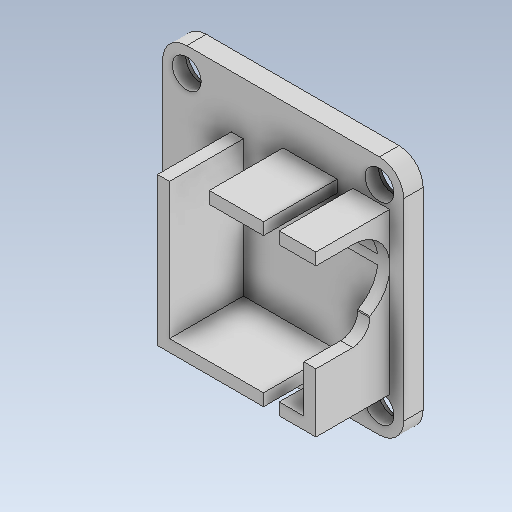
# Autodesk Inventor part: apoio servo
Saved by Autodesk Inventor 2020 (Build 240168000, 168)
## iProperties
Created: 2020-04-22
Part Number: apoio servo
Material: Genérico
Document SubType Name: Modeling
Designer: gi-se
Density: 1 g/cm^3
Appearance: Padrão
Author: gi-se
Autodesk Inventor part; units mm, degrees
ref_plane "YZ Plane" through (0, 0, 0) normal (1, 0, 0) x (0, 1, 0)
ref_plane "XZ Plane" through (0, 0, 0) normal (0, 1, 0) x (-1, 0, 0)
ref_plane "XY Plane" through (0, 0, 0) normal (0, 0, 1) x (1, 0, 0)
sketch "Esboço1" plane through (0, 0, 0) normal (0, 0, 1) x (1, 0, 0)
  circle A0 centre (0, 51.901) radius 2.4 projected
  circle A1 centre (0, 19.901) radius 2.4 projected
  circle A2 centre (-32, 19.901) radius 2.4 projected
  line L0 (-36, 3.901) -> (-36, 51.901) projected
  circle A3 centre (0, 19.901) radius 4
  circle A4 centre (0, 51.901) radius 4
  circle A5 centre (-32, 19.901) radius 4
  line L1 (-36, 15.901) -> (0, 15.901)
  line L2 (4, 19.901) -> (4, 51.901)
  line L3 (0, 55.901) -> (-36, 55.901)
  line L4 (-36, 55.901) -> (-36, 15.901)
  circle A6 centre (-32, 51.901) radius 4
  circle A7 centre (-32, 51.901) radius 2.4 projected
  point P0 (0, 0)
  point P1 (-36, 19.901)
  point P2 (-32, 15.901)
  point P3 (-32, 55.901)
  dimension "d0" = 8
  dimension "d1" = 8
  dimension "d2" = 8
  dimension "d12" = 8
  constraints: 8 end point, 4 centre point, 4 point on circle, 3 coincident, 2 parallel, 1 horizontal, 1 perpendicular, 1 point on line
  measures "d0" diameter of A3
  measures "d1" diameter of A4
  measures "d2" diameter of A5
  measures "d12" diameter of A6
extrude "Extrusão1" add sketch "Esboço1" along normal blind 3.25 contours L0 A6 L3 A4 L2 A3 L1 A5 | A5 | A6 | A3 | A4
sketch "Esboço2" plane through (0, 0, 3.25) normal (0, 0, 1) x (1, 0, 0)
  arc A0 (-22.6, 24.751) -> (-22.45, 24.601) centre (-22.45, 24.751) ccw projected
  line L0 (-0.3, 39.0723) -> (-0.3, 24.751) projected
  line L1 (-4.4, 47.201) -> (-0.45, 47.201) projected
  line L2 (-0.3, 24.601) -> (-0.3, 47.201)
  line L3 (-22.6, 47.201) -> (-22.6, 24.601)
  line L4 (1.7, 49.201) -> (1.7, 22.601)
  line L5 (-24.6, 22.601) -> (-24.6, 47.201)
  line L6 (-22.6, 47.201) -> (-24.6, 47.201)
  line L7 (-7, 49.201) -> (-7, 47.201)
  line L8 (-4.4, 49.201) -> (-4.4, 47.201)
  line L9 (-4.4, 24.601) -> (-4.4, 22.601)
  line L10 (-7, 24.601) -> (-7, 22.601)
  line L11 (-22.6, 24.601) -> (-7, 24.601)
  line L12 (-4.4, 24.601) -> (-0.3, 24.601)
  line L13 (1.7, 22.601) -> (-4.4, 22.601)
  line L14 (-7, 22.601) -> (-24.6, 22.601)
  line L15 (-16, 49.201) -> (-7, 49.201)
  line L16 (-4.4, 49.201) -> (1.7, 49.201)
  line L17 (-0.3, 47.201) -> (-4.4, 47.201)
  line L18 (-7, 47.201) -> (-16, 47.201)
  line L19 (-16, 47.201) -> (-16, 49.201)
  point P0 (0, 0)
  constraints: 36 end point, 10 parallel, 10 perpendicular, 4 point on line, 2 horizontal
extrude "Extrusão2" add sketch "Esboço2" along normal blind 12.25 contours L3 L11 L10 L14 L5 L6 | L2 L17 L1 L8 L16 L4 L13 L9 L12 L0 | L7 L18 L19 L15
sketch "Esboço3" plane through (1.7, 22.601, 3.25) normal (1, 0, 0) x (0, 0, -1)
  arc A0 (-6.15, 9.8) -> (-3.3, 12.65) centre (-6.15, 12.65) ccw
  line L0 (-3.3, 12.8939) -> (-3.3, 12.65)
  line L1 (-6.15, 9.8) -> (-12.25, 9.8)
  line L2 (-12.25, 24.6) -> (-12.25, 0) projected
  line L3 (0, 24.6) -> (-12.25, 24.6) projected
  line L4 (-6.15, 24.6) -> (-12.25, 24.6)
  arc A1 (-3.3, 12.8939) -> (-6.15, 24.6) centre (-6.15, 18.4) ccw
  point P0 (3.25, -22.601)
  constraints: 6 end point, 4 point on circle, 2 centre point, 2 point on line, 1 collinear, 1 horizontal, 1 tangent, 1 vertical, 6 other
extrude "Extrusão3" cut sketch "Esboço3" against normal blind 12.25
sketch "Esboço4" plane through (0, 0, 0) normal (0, 0, -1) x (-1, 0, 0)
  circle A0 centre (0, 19.901) radius 2.4 projected
  circle A1 centre (32, 19.901) radius 2.4 projected
  circle A2 centre (0, 51.901) radius 2.4 projected
  circle A3 centre (32, 51.901) radius 2.4 projected
  circle A4 centre (32, 51.901) radius 3.1 projected
  circle A5 centre (0, 51.901) radius 3.1 projected
  circle A6 centre (0, 19.901) radius 3.1 projected
  circle A7 centre (32, 19.901) radius 3.1 projected
  point P0 (0, 0)
extrude "Extrusão4" cut sketch "Esboço4" against normal blind 1
